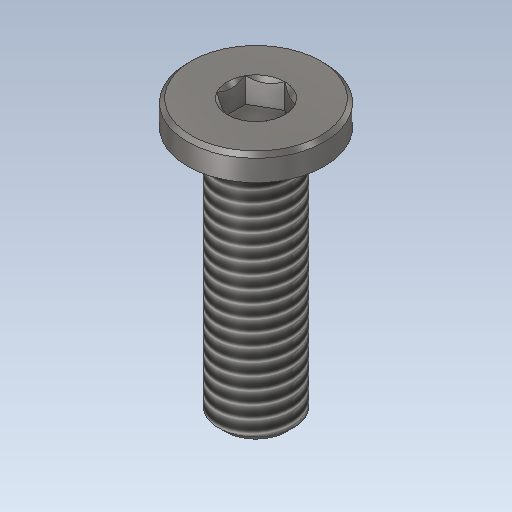
# Autodesk Inventor part: 48-03A1
Saved by Autodesk Inventor 2021 (Build 250183000, 183)
## iProperties
Created: 2016-07-02
Part Number: 48-03A1
Material: Stainless Steel
Document SubType Name: Modeling
Designer: Bradley
Density: 8 g/cm^3
Appearance: Semi-Polished
Description: SCM4006-3H3
Stock Number: 80110
Manager: Bradley
Company: Zetta & Zepto Technology
Author: Bradley
Autodesk Inventor part; units mm, degrees
ref_plane "YZ Plane" through (0, 0, 0) normal (1, 0, 0) x (0, 1, 0)
ref_plane "XZ Plane" through (0, 0, 0) normal (0, 1, 0) x (-1, 0, 0)
ref_plane "XY Plane" through (0, 0, 0) normal (0, 0, 1) x (1, 0, 0)
sketch "Sketch1" plane through (0, 0, 0) normal (0, 0, 1) x (1, 0, 0)
  line L0 (0, 5.5) -> (0, -5.5)
  line L1 (0, -5.5) -> (1.25, -5.5)
  line L2 (1.25, -5.5) -> (1.5, -5.25)
  line L3 (1.5, -5.25) -> (1.5, 4.4)
  line L4 (1.6, 4.5) -> (2.75, 4.5)
  line L5 (2.75, 4.5) -> (2.75, 5.35)
  line L6 (2.6, 5.5) -> (0, 5.5)
  arc A0 (1.6, 4.5) -> (1.5, 4.4) centre (1.6, 4.4) ccw
  line L7 (2.6, 5.5) -> (2.75, 5.35)
  point P0 (0, 0)
  point P1 (2.75, 5.5)
  point P2 (0, 0)
  dimension "d0" = 5.5
  dimension "d1" = 1
  dimension "d3" = 3
  dimension "d4" = 3.2
  dimension "d5" = 135
  dimension "d6" = 0.25
  dimension "d7" = 10
  dimension "d18" = 0.15
  dimension "d22" = 0.15
  constraints: 18 end point, 4 perpendicular, 4 point on line, 2 point on circle, 2 tangent, 1 centre point, 1 coincident, 1 midpoint, 1 parallel, 1 vertical
  measures "d0" diameter of L5 L0
  measures "d1" distance of L4.end point (2.75, 5.5)
  measures "d3" diameter of L3 L0
  measures "d4" diameter of L4.start L0
  measures "d5" angle of L3 L2
  measures "d6" horizontal distance of L1.end L2.end
  measures "d7" distance between parallel lines of L1 L4
  measures "d18" distance of L6.start point (2.75, 5.5)
  measures "d22" horizontal distance of L6.start L5.end
revolve "Revolution1" add sketch "Sketch1" angle 360 about axis through (0, 5.5, 0) along (0, -1, 0)
sketch "Sketch2" plane through (0, 5.5, 0) normal (0, 1, 0) x (1, 0, 0)
  line L0 (0, -1.1547) -> (-1, -0.5774)
  line L1 (-1, -0.5774) -> (-1, 0.5774)
  line L2 (-1, 0.5774) -> (0, 1.1547)
  line L3 (0, 1.1547) -> (1, 0.5774)
  line L4 (1, 0.5774) -> (1, -0.5774)
  line L5 (1, -0.5774) -> (0, -1.1547)
  point P0 (0, 0)
  point P1 (0, 0)
  dimension "d11" = 2
  constraints: 12 end point, 1 coincident, 1 vertical, 13 other
  measures "d11" distance between parallel lines of L4 L1
extrude "Extrusion1" cut sketch "Sketch2" against normal blind 1
thread "Thread1" size "M3x0.5" class "6g" standard "ANSI Metric M Profile" full length
sketch "Sketch3" plane through (0, 0, 0) normal (1, 0, 0) x (0, 1, 0)
  line L0 (5.5, 1.1547) -> (5.5, 0.5774) projected
  line L1 (5.5, 1.1547) -> (5, 0.6547)
  line L2 (5, 0.6547) -> (5.5, 0.6547)
  line L3 (5.5, 0.6547) -> (5.5, 1.1547)
  line L4 (-0.9, 0) -> (5.4, 0) projected
  point P0 (0, 0)
  dimension "d16" = 0.5
  constraints: 6 end point, 3 perpendicular
  measures "d16" distance of L2.end L0.start
revolve "Revolution2" cut sketch "Sketch3" angle 360 about axis through (0, -10, 0) along (0, 1, 0)
equation "\"d22\" = d18"
body "Solid1"
